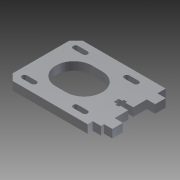
# Autodesk Inventor part: carro x lado motor pieza 5 soporte nema
Saved by Autodesk Inventor 2012 (Build 160160000, 160)
## iProperties
Created: 2014-12-17
Part Number: carro x lado motor pieza 5 soporte nema
Material: Default
Document SubType Name: Modeling
Designer: PRINCIPAL
Density: 1 g/cm^3
Author: PRINCIPAL
Autodesk Inventor part; units mm, degrees
ref_plane "YZ Plane" through (0, 0, 0) normal (1, 0, 0) x (0, 1, 0)
ref_plane "XZ Plane" through (0, 0, 0) normal (0, 1, 0) x (-1, 0, 0)
ref_plane "XY Plane" through (0, 0, 0) normal (0, 0, 1) x (1, 0, 0)
sketch "Boceto1" plane through (0, 0, 0) normal (0, 0, 1) x (1, 0, 0)
  line L0 (1.2797, 34.95) -> (7.0205, 34.95)
  arc A0 (7.0205, 34.95) -> (7.0205, 38.05) centre (7.0205, 36.5) ccw
  line L1 (7.0205, 38.05) -> (1.2797, 38.05)
  arc A1 (1.2797, 38.05) -> (-0.2703, 36.5) centre (1.2797, 36.5) ccw
  arc A2 (-0.2703, 36.5) -> (1.2797, 34.95) centre (1.2797, 36.5) ccw
  line L2 (7.0205, 7.05) -> (1.2797, 7.05)
  arc A3 (1.2797, 7.05) -> (-0.2703, 5.5) centre (1.2797, 5.5) ccw
  arc A4 (-0.2703, 5.5) -> (1.2797, 3.95) centre (1.2797, 5.5) ccw
  line L3 (1.2797, 3.95) -> (7.0205, 3.95)
  arc A5 (7.0205, 3.95) -> (7.0205, 7.05) centre (7.0205, 5.5) ccw
  arc A6 (38.0205, 34.95) -> (38.0205, 38.05) centre (38.0205, 36.5) ccw
  line L4 (38.0205, 38.05) -> (32.2797, 38.05)
  arc A7 (32.2797, 38.05) -> (30.7297, 36.5) centre (32.2797, 36.5) ccw
  arc A8 (30.7297, 36.5) -> (32.2797, 34.95) centre (32.2797, 36.5) ccw
  line L5 (32.2797, 34.95) -> (38.0205, 34.95)
  arc A9 (15.751, 31.95) -> (4.801, 21) centre (15.751, 21) ccw
  arc A10 (4.801, 21) -> (15.751, 10.05) centre (15.751, 21) ccw
  line L6 (15.751, 10.05) -> (21.9491, 10.05)
  arc A11 (21.9491, 10.05) -> (21.9491, 31.95) centre (21.9491, 21) ccw
  line L7 (21.9491, 31.95) -> (15.751, 31.95)
  line L8 (38.0205, 7.05) -> (32.2797, 7.05)
  arc A12 (32.2797, 7.05) -> (30.7297, 5.5) centre (32.2797, 5.5) ccw
  arc A13 (30.7297, 5.5) -> (32.2797, 3.95) centre (32.2797, 5.5) ccw
  line L9 (32.2797, 3.95) -> (38.0205, 3.95)
  arc A14 (38.0205, 3.95) -> (38.0205, 7.05) centre (38.0205, 5.5) ccw
  line L10 (45.2649, -0.2) -> (45.2649, 2.9451)
  line L11 (45.2649, 2.9451) -> (50.2083, 2.9451)
  line L12 (50.2083, 2.9451) -> (50.2083, 4.8)
  line L13 (50.2083, 4.8) -> (55.2083, 4.8)
  line L14 (55.2083, 4.8) -> (55.2083, 11.2)
  line L15 (55.2083, 11.2) -> (50.2083, 11.2)
  line L16 (50.2083, 11.2) -> (50.2083, 19.45)
  line L17 (50.2083, 19.45) -> (45.3976, 19.45)
  line L18 (45.3976, 19.45) -> (45.3976, 18.45)
  line L19 (45.3976, 18.45) -> (43.3976, 18.45)
  line L20 (43.3976, 18.45) -> (43.3976, 19.45)
  line L21 (43.3976, 19.45) -> (41.3976, 19.45)
  line L22 (41.3976, 19.45) -> (41.3976, 22.55)
  line L23 (41.3976, 22.55) -> (43.3976, 22.55)
  line L24 (43.3976, 22.55) -> (43.3976, 23.55)
  line L25 (43.3976, 23.55) -> (45.3976, 23.55)
  line L26 (45.3976, 23.55) -> (45.3976, 22.55)
  line L27 (45.3976, 22.55) -> (50.2083, 22.55)
  line L28 (50.2083, 22.55) -> (50.2083, 30.8)
  line L29 (50.2083, 30.8) -> (55.2083, 30.8)
  line L30 (55.2083, 30.8) -> (55.2083, 37.2)
  line L31 (55.2083, 37.2) -> (50.2083, 37.2)
  line L32 (50.2083, 37.2) -> (50.2083, 42.2)
  line L33 (50.2083, 42.2) -> (-0.0828, 42.2)
  line L34 (-0.0828, 42.2) -> (-4.2, 38.0828)
  line L35 (-4.2, 38.0828) -> (-4.2, 3.9172)
  line L36 (-4.2, 3.9172) -> (-0.0828, -0.2)
  line L37 (-0.0828, -0.2) -> (45.2649, -0.2)
  point P0 (0, 0)
  constraints: 76 end point, 30 point on circle, 15 centre point
extrude "Extrusión1" add sketch "Boceto1" along normal blind 5
